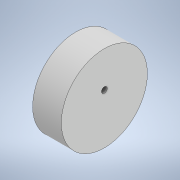
# Autodesk Inventor part: 711116
Saved by Autodesk Inventor 2022 (Build 260153000, 153)
## iProperties
Created: 2021-10-21
Part Number: 711116
Material: Типовые
Document SubType Name: Modeling
Designer: RaNSiD
Density: 1 g/cm^3
Appearance: По умолчанию
Author: RaNSiD
Autodesk Inventor part; units mm, degrees
ref_plane "YZ Plane" through (0, 0, 0) normal (1, 0, 0) x (0, 1, 0)
ref_plane "XZ Plane" through (0, 0, 0) normal (0, 1, 0) x (-1, 0, 0)
ref_plane "XY Plane" through (0, 0, 0) normal (0, 0, 1) x (1, 0, 0)
sketch "Эскиз1" plane through (0, 0, 0) normal (0, 0, 1) x (1, 0, 0)
  line L0 (0, 0) -> (20, 0)
  line L1 (20, 0) -> (20, 30)
  line L2 (20, 30) -> (0, 30)
  line L3 (0, 30) -> (0, 0)
  dimension "d0" = 20
  dimension "d1" = 30
  constraints: 8 end point, 2 parallel, 1 horizontal, 1 perpendicular
  measures "d0" distance of L2.end L1.end
  measures "d1" distance of L1.end L0.end
revolve "Вращение1" add sketch "Эскиз1" angle 360 about axis through (0, 0, 0) along (1, 0, 0)
sketch "Эскиз2" plane through (0, 0, 0) normal (-1, 0, 0) x (0, 0, 1)
  circle A0 centre (0, 5) radius 2
  point P0 (0, 0)
  dimension "d3" = 4
  dimension "d4" = 5
  constraints: 1 centre point, 1 vertical alignment
  measures "d3" diameter of A0
  measures "d4" distance of point (0, 0) A0.centre
extrude "Выдавливание1" cut sketch "Эскиз2" against normal blind 20
sketch "Эскиз3" plane through (0, 0, 0) normal (0, 0, 1) x (1, 0, 0)
  line L0 (0, 3) -> (0, 7) projected
  line L1 (0, -30) -> (0, 30) construction
  line L2 (0, 22) -> (4.5, 22)
  line L3 (0, 23.0379) -> (4.5, 24.5)
  line L4 (4.5, 24.5) -> (4.5, 22)
  line L5 (0, 0) -> (20, 0)
  line L6 (20, -30) -> (20, 30) construction
  line L7 (0, 22) -> (0, 23.0379)
  dimension "d7" = 4.5
  dimension "d8" = 22
  dimension "d10" = 72
  dimension "d12" = 2.5
  constraints: 10 end point, 2 coincident, 2 point on line, 1 collinear, 1 horizontal, 1 midpoint, 1 vertical
  measures "d7" distance of L2.start L2.end
  measures "d8" distance of L5.start L2.start
  measures "d10" angle of L3 L4
  measures "d12" distance of L3.end L2.end
revolve "Вращение2" cut sketch "Эскиз3" angle 360 about axis through (0, 22, 0) along (1, 0, 0)
mirror "Зеркальное отражение1" about plane through (0, 0, 0) normal (0, 1, 0) of "Вращение2"
